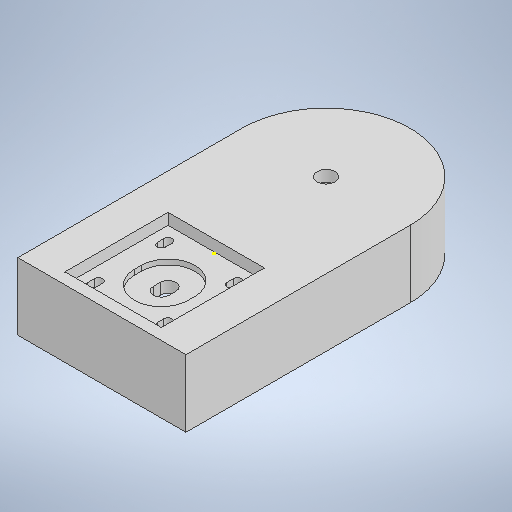
# Autodesk Inventor part: SCARA base
Saved by Autodesk Inventor 2025.2 (Build 292293000, 293)
## iProperties
Created: 2025-01-25
Part Number: SCARA base
Material: Generic
Document SubType Name: Modeling
Designer: caomi
Density: 1 g/cm^3
Appearance: Default
Author: caomi
Autodesk Inventor part; units mm, degrees
ref_plane "YZ Plane" through (0, 0, 0) normal (1, 0, 0) x (0, 1, 0)
ref_plane "XZ Plane" through (0, 0, 0) normal (0, 1, 0) x (-1, 0, 0)
ref_plane "XY Plane" through (0, 0, 0) normal (0, 0, 1) x (1, 0, 0)
sketch "Sketch1" plane through (0, 0, 0) normal (0, 1, 0) x (-1, 0, 0)
  line L0 (-37.5, -50) -> (37.5, -50)
  line L1 (37.5, -50) -> (37.5, 50)
  line L2 (37.5, 50) -> (-37.5, 50)
  line L3 (-37.5, 50) -> (-37.5, -50)
  line L4 (-37.5, -50) -> (37.5, 50) construction
  line L5 (37.5, -50) -> (-37.5, 50) construction
  circle A0 centre (0, -50) radius 37.5
  point P0 (0, 0)
  point P1 (-37.5, -50)
  dimension "d2" = 75
  dimension "d4" = 100
  constraints: 12 end point, 3 midpoint, 2 parallel, 1 horizontal, 1 perpendicular, 3 other
  measures "d2" distance of L1.end L2.end
  measures "d4" distance of L0.end L1.end
extrude "Extrusion1" add sketch "Sketch1" along normal blind 30
sketch "Sketch2" plane through (0, 30, 0) normal (0, 1, 0) x (1, 0, 0)
  line L0 (-15.5, -39) -> (-15.5, -36) construction
  line L1 (-13.7, -39) -> (-13.7, -36)
  line L2 (-17.3, -36) -> (-17.3, -39)
  arc A0 (-17.3, -39) -> (-13.7, -39) centre (-15.5, -39) ccw
  arc A1 (-13.7, -36) -> (-17.3, -36) centre (-15.5, -36) ccw
  line L3 (-15.5, -8) -> (-15.5, -5) construction
  line L4 (-13.7, -8) -> (-13.7, -5)
  line L5 (-17.3, -5) -> (-17.3, -8)
  arc A2 (-17.3, -8) -> (-13.7, -8) centre (-15.5, -8) ccw
  arc A3 (-13.7, -5) -> (-17.3, -5) centre (-15.5, -5) ccw
  line L6 (15.5, -39) -> (15.5, -36) construction
  line L7 (17.3, -39) -> (17.3, -36)
  line L8 (13.7, -36) -> (13.7, -39)
  arc A4 (13.7, -39) -> (17.3, -39) centre (15.5, -39) ccw
  arc A5 (17.3, -36) -> (13.7, -36) centre (15.5, -36) ccw
  line L9 (15.5, -8) -> (15.5, -5) construction
  line L10 (17.3, -8) -> (17.3, -5)
  line L11 (13.7, -5) -> (13.7, -8)
  arc A6 (13.7, -8) -> (17.3, -8) centre (15.5, -8) ccw
  arc A7 (17.3, -5) -> (13.7, -5) centre (15.5, -5) ccw
  line L12 (0, -20.5) -> (0, -23.5) construction
  line L13 (-12, -20.5) -> (-12, -23.5)
  line L14 (12, -23.5) -> (12, -20.5)
  arc A8 (12, -20.5) -> (-12, -20.5) centre (0, -20.5) ccw
  arc A9 (-12, -23.5) -> (12, -23.5) centre (0, -23.5) ccw
  line L15 (-15.5, -6.5) -> (15.5, -37.5) construction
  line L16 (-15.5, -37.5) -> (15.5, -6.5) construction
  line L17 (21.5, 1) -> (-21.5, 1)
  line L18 (-21.5, 1) -> (-21.5, -45)
  line L19 (-21.5, -45) -> (21.5, -45)
  line L20 (21.5, -45) -> (21.5, 1)
  line L21 (21.5, 1) -> (-21.5, -45) construction
  line L22 (-21.5, 1) -> (21.5, -45) construction
  line L23 (-37.5, -50) -> (37.5, -50) projected
  line L24 (0, -20.5) -> (0, -23.5) construction
  line L25 (-3.5, -20.5) -> (-3.5, -23.5)
  line L26 (3.5, -23.5) -> (3.5, -20.5)
  arc A10 (3.5, -20.5) -> (-3.5, -20.5) centre (0, -20.5) ccw
  arc A11 (-3.5, -23.5) -> (3.5, -23.5) centre (0, -23.5) ccw
  point P0 (0, 0)
  point P1 (0, -22)
  point P2 (0, -22)
  dimension "d18" = 1.8
  dimension "d20" = 3
  dimension "d45" = 12
  dimension "d48" = 31
  dimension "d49" = 31
  dimension "d50" = 43
  dimension "d51" = 46
  dimension "d52" = 5
  dimension "d53" = 3.5
  constraints: 64 end point, 24 point on circle, 24 tangent, 12 centre point, 9 midpoint, 8 parallel, 6 vertical, 5 equal length, 4 vertical alignment, 3 equal radius, 2 horizontal alignment, 1 coincident, 1 horizontal, 1 perpendicular
  measures "d18" radius of A1
  measures "d20" distance of L2.start L2.end
  measures "d45" radius of A9
  measures "d48" distance from line of L16.start L6
  measures "d49" distance of L16.start L15.start
  measures "d50" distance of L18.end L19.end
  measures "d51" distance of L17.end L18.end
  measures "d52" distance between parallel lines of L19 L23
  measures "d53" radius of A11
extrude "Extrusion2" cut sketch "Sketch2" against normal blind 5 contours A0 L2 A1 L1 | A2 L5 A3 L4 | A4 L8 A5 L7 | A6 L11 A7 L10 | A8 L14 A9 L13 | L20 L19 L18 L17 | A10 L26 A11 L25
extrude "Extrusion3" cut sketch "Sketch2" against normal blind 2.3 from surface at -5 contours A8 L14 A9 L13 | A10 L26 A11 L25
shell "Shell1" thickness 5 removed faces 1 at (12.5, 0, 16.6667)
extrude "Extrusion4" cut sketch "Sketch2" against normal up to surface (30 mm away) contours A0 L2 A1 L1 | A2 L5 A3 L4 | A4 L8 A5 L7 | A6 L11 A7 L10 | A10 L26 A11 L25
sketch "Sketch6" plane through (0, 25, -50) normal (0, -1, 0) x (1, 0, 0)
  circle A0 centre (0, 0) radius 12.375
  circle A1 centre (0, 0) radius 16.875
  circle A2 centre (0, 0) radius 22.5
  arc A3 (-32.5, 0) -> (32.5, 0) centre (0, 0) ccw projected
  point P0 (0, 50)
  dimension "d29" = 45
  constraints: 3 centre point, 2 concentric, 1 coincident
  measures "d29" diameter of A2
extrude "Extrusion7" add sketch "Sketch6" along normal blind 7 contours A1
sketch "Sketch9" plane through (0, 30, 0) normal (0, 1, 0) x (1, 0, 0)
  circle A0 centre (0, 50) radius 4
  circle A1 centre (0, 50) radius 17.5
  arc A2 (37.5, 50) -> (-37.5, 50) centre (0, 50) ccw projected
  point P0 (0, 0)
  dimension "d39" = 8
  dimension "d40" = 35
  constraints: 2 centre point, 1 coincident, 1 concentric
  measures "d39" diameter of A0
  measures "d40" diameter of A1
extrude "Extrusion11" cut sketch "Sketch9" against normal up to surface (5 mm away) contours A0
sketch "Sketch10" plane through (0, 25, -50) normal (0, -1, 0) x (1, 0, 0)
  point P0 (0, 50)
equation "\"d51\" = d50 + d20"
body "Solid1"
